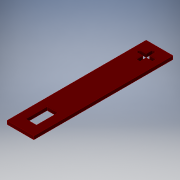
# Autodesk Inventor part: Brazo_Superior
Saved by Autodesk Inventor 2019 (Build 230136000, 136)
## iProperties
Created: 2020-02-09
Part Number: Brazo_Superior
Material: Generic
Document SubType Name: Modeling
Designer: Omar
Density: 1 g/cm^3
Appearance: Default
Author: Omar
Autodesk Inventor part; units mm, degrees
ref_plane "YZ Plane" through (0, 0, 0) normal (1, 0, 0) x (0, 1, 0)
ref_plane "XZ Plane" through (0, 0, 0) normal (0, 1, 0) x (-1, 0, 0)
ref_plane "XY Plane" through (0, 0, 0) normal (0, 0, 1) x (1, 0, 0)
sketch "Sketch1" plane through (0, 0, 0) normal (0, 1, 0) x (-1, 0, 0)
  line L0 (-5, 10) -> (5, 10)
  line L1 (5, 10) -> (5, -10)
  line L2 (5, -10) -> (-5, -10)
  line L3 (-5, -10) -> (-5, 10)
  line L4 (-5, 10) -> (5, -10) construction
  line L5 (5, 10) -> (-5, -10) construction
  line L6 (12.5, 20) -> (-12.5, 20)
  line L7 (-12.5, 20) -> (-12.5, -110)
  line L8 (-12.5, -110) -> (12.5, -110)
  line L9 (12.5, -110) -> (12.5, 20)
  line L10 (1.59, -105) -> (-1.59, -105)
  line L11 (-1.59, -105) -> (-1.59, -90)
  line L12 (-1.59, -90) -> (1.59, -90)
  line L13 (1.59, -90) -> (1.59, -105)
  line L14 (1.59, -105) -> (-1.59, -90) construction
  line L15 (-1.59, -105) -> (1.59, -90) construction
  line L16 (7.5, -95.91) -> (-7.5, -95.91)
  line L17 (-7.5, -95.91) -> (-7.5, -99.09)
  line L18 (-7.5, -99.09) -> (7.5, -99.09)
  line L19 (7.5, -99.09) -> (7.5, -95.91)
  line L20 (7.5, -95.91) -> (-7.5, -99.09) construction
  line L21 (-7.5, -95.91) -> (7.5, -99.09) construction
  point P0 (0, 0)
  point P1 (0, 0)
  point P2 (0, 0)
  point P3 (0, -97.5)
  dimension "d24" = 10
  dimension "d25" = 20
  dimension "d26" = 25
  dimension "d27" = 130
  dimension "d28" = 20
  dimension "d29" = 12.5
  dimension "d37" = 3.18
  dimension "d38" = 15
  dimension "d39" = 15
  dimension "d40" = 3.18
  dimension "d41" = 12.5
  dimension "d42" = 12.5
  constraints: 44 end point, 8 parallel, 7 midpoint, 4 horizontal, 4 perpendicular, 1 coincident
  measures "d24" distance of L1.end L2.end
  measures "d25" distance of L0.end L1.end
  measures "d26" distance of L8.end L7.end
  measures "d27" distance of L8.end L6.start
  measures "d28" distance from line of L6 point (0, 0)
  measures "d29" distance from line of L9 point (0, 0)
  measures "d37" distance of L11.end L12.end
  measures "d38" distance of L10.end L11.end
  measures "d39" distance of L18.end L17.end
  measures "d40" distance of L17.end L16.end
  measures "d41" distance from line of L9 point (0, -97.5)
  measures "d42" distance from line of L8 point (0, -97.5)
extrude "Extrusion3" add sketch "Sketch1" along normal blind 3.18
body "Solid3"
